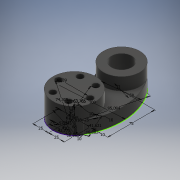
# Autodesk Inventor part: Кронштейн
Saved by Autodesk Inventor 2018 (Build 220112000, 112)
## iProperties
Created: 2020-04-13
Part Number: Кронштейн
Material: Полиацеталь, черный
Document SubType Name: ЛистМат
Designer: Alena Oparina
Density: 1.425 g/cm^3
Appearance: Гладкая - черная
Sheet Metal Rule: По умолчанию
Author: Alena Oparina
Autodesk Inventor part; units mm, degrees
ref_plane "YZ Plane" through (0, 0, 0) normal (1, 0, 0) x (0, 1, 0)
ref_plane "XZ Plane" through (0, 0, 0) normal (0, 1, 0) x (-1, 0, 0)
ref_plane "XY Plane" through (0, 0, 0) normal (0, 0, 1) x (1, 0, 0)
sketch "Эскиз1" plane through (0, 0, 0) normal (0, 0, 1) x (1, 0, 0)
  circle A0 centre (0, 0) radius 34
  circle A1 centre (0, 75) radius 29
  circle A2 centre (0, 75) radius 16
  arc A3 (29.9201, -16.149) -> (23.364, 92.1791) centre (-57.2016, 32.9408) ccw
  arc A4 (-24.1868, 23.8956) -> (-24.1868, 59) centre (-61.6709, 41.4478) ccw
  circle A5 centre (-25, 0) radius 5
  circle A6 centre (25, 0) radius 5
  circle A7 centre (-12.5, 21.6506) radius 5
  circle A8 centre (12.5, 21.6506) radius 5
  circle A9 centre (-12.5, -21.6506) radius 5
  circle A10 centre (12.5, -21.6506) radius 5
  point P0 (-24.5501, 23.5222)
  dimension "d2" = 58
  dimension "d3" = 32
  dimension "d7" = 100
  dimension "d18" = 41.3901
  dimension "d29" = 10
  dimension "d30" = 10
  dimension "d31" = 10
  dimension "d32" = 10
  dimension "d33" = 10
  dimension "d34" = 10
  dimension "d35" = 68
  dimension "d36" = 25
  dimension "d37" = 95.094
  dimension "d38" = 25
  dimension "d39" = 25
  dimension "d40" = 75
  dimension "d41" = 25
  dimension "d42" = 25
  dimension "d43" = 63.7652
  dimension "d44" = 63.7652
  dimension "d45" = 25
  dimension "d46" = 74.3049
  dimension "d47" = 16.8819
  dimension "d48" = 41.6206
  dimension "d49" = 18.2682
  dimension "d50" = 56.8179
  dimension "d51" = 42.7753
  dimension "d52" = 67.3855
  dimension "d53" = 57.2451
  constraints: 11 centre point, 10 point on circle, 2 coincident, 1 tangent
  measures "d2" diameter of A1
  measures "d3" diameter of A2
  measures "d7" radius of A3
  measures "d18" radius of A4
  measures "d29" diameter of A5
  measures "d30" diameter of A6
  measures "d31" diameter of A7
  measures "d32" diameter of A8
  measures "d33" diameter of A9
  measures "d34" diameter of A10
  measures "d35" diameter of A0
  measures "d36" distance of A6.centre point (0, 0)
  measures "d37" distance of A1.start point (0, 0)
  measures "d38" distance of A8.centre point (0, 0)
  measures "d39" distance of A10.centre point (0, 0)
  measures "d40" distance of A1.centre point (0, 0)
  measures "d41" distance of A7.centre point (0, 0)
  measures "d42" distance of A9.centre point (0, 0)
  measures "d43" distance of A4.end point (0, 0)
  measures "d44" distance of A1.end point (0, 0)
  measures "d45" distance of A5.centre point (0, 0)
  measures "d46" distance of A4.centre point (0, 0)
  measures "d47" distance of A6.centre A0.start
  measures "d48" distance of A8.centre A0.start
  measures "d49" distance of A10.centre A0.start
  measures "d50" distance of A7.centre A0.start
  measures "d51" distance of A9.centre A0.start
  measures "d52" distance of A0.end A0.start
  measures "d53" distance of A5.centre A0.start
extrude "Выдавливание3" add sketch "Эскиз1" along normal blind 40 contours A0 | A1
extrude "Выдавливание4" cut sketch "Эскиз1" along normal blind 20 contours A0 A4 A1 A3
extrude "Выдавливание5" add sketch "Эскиз1" along normal blind 20 contours A0 A4 A1 A3
equation "\"Радиус_гибки\" = Толщина"
equation "\"Ширина_просечки\" = Толщина"
equation "\"Глубина_просечки\" = 0.5 * Толщина"
equation "\"Размер_просечки\" = 4 * Толщина"
equation "\"Мин_остаток\" = 2 * Толщина"
equation "\"Радиус_перехода\" = Радиус_гибки"
equation "\"Радиус_Якоби\" = Толщина"
equation "\"Размер_зазора\" = Толщина"
equation "\"Толщина\" = 3.048"
